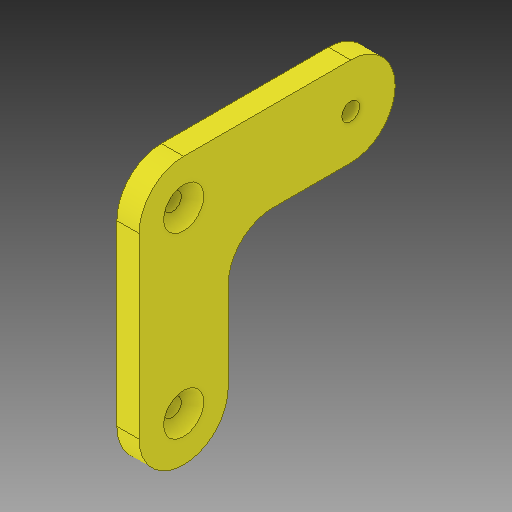
# Autodesk Inventor part: upper anchor
Saved by Autodesk Inventor 2017 SP1 (Build 210196100, 196)
## iProperties
Created: 2018-01-21
Part Number: upper anchor
Material: Aluminum 6061
Document SubType Name: Modeling
Designer: Ben
Density: 2.7 g/cm^3
Appearance: Canary
Mass: 49.892 g
Surface Area: 78.5017 cm^2
Volume: 18.4785 cm^3
Author: Ben
Autodesk Inventor part; units mm, degrees
ref_plane "YZ Plane" through (0, 0, 0) normal (1, 0, 0) x (0, 1, 0)
ref_plane "XZ Plane" through (0, 0, 0) normal (0, 1, 0) x (-1, 0, 0)
ref_plane "XY Plane" through (0, 0, 0) normal (0, 0, 1) x (1, 0, 0)
sketch "Sketch1" plane through (0, 0, 0) normal (1, 0, 0) x (0, 1, 0)
  circle A0 centre (0, 0) radius 2.54
  circle A1 centre (-50.8, 0) radius 2.54
  circle A2 centre (0, -47.625) radius 2.54
  line L0 (0, 0) -> (-50.8, 0) construction
  line L1 (0, -47.625) -> (0, 0) construction
  arc A3 (-50.8, 12.7) -> (-50.8, -12.7) centre (-50.8, 0) ccw
  arc A4 (12.7, 0) -> (0, 12.7) centre (0, 0) ccw
  arc A5 (-12.7, -47.625) -> (12.7, -47.625) centre (0, -47.625) ccw
  arc A6 (-12.7, -25.4) -> (-25.4, -12.7) centre (-25.4, -25.4) ccw
  line L2 (0, 12.7) -> (-50.8, 12.7)
  line L3 (12.7, 0) -> (12.7, -47.625)
  line L4 (-12.7, -47.625) -> (-12.7, -25.4)
  line L5 (-25.4, -12.7) -> (-50.8, -12.7)
  dimension "d0" = 5.08
  dimension "d1" = 50.8
  dimension "d2" = 47.625
  dimension "d3" = 25.4
  constraints: 12 end point, 8 point on circle, 8 tangent, 7 centre point, 4 coincident, 4 equal radius, 2 perpendicular, 1 horizontal, 1 parallel, 1 vertical
  measures "d0" diameter of A0
  measures "d1" distance of L0.end point (0, 0)
  measures "d2" distance of point (0, 0) L1.start
  measures "d3" distance between parallel lines of L2 L5
extrude "Extrusion1" add sketch "Sketch1" along normal blind 6.35
chamfer "Chamfer1" distance 3.175 angle 45 2 edges at (6.35, -2.54, 0) (6.35, -53.34, 0)
body "Solid1"
